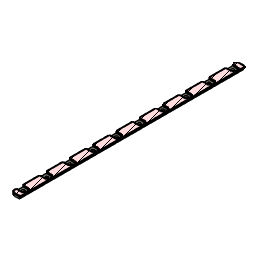
voron_v0_new_nut_holder (Autodesk Fusion 360 design; units mm, degrees)
Autodesk Fusion 360 part; units mm, degrees
sketch "Sketch1" plane through (0, 0, 0) normal (0, 0, 1) x (1, 0, 0)
  circle A0 centre (0, 0) radius 1.25
  line L0 (2.45, 0) -> (1.225, 2.1218)
  line L1 (1.225, 2.1218) -> (-1.225, 2.1218)
  line L2 (-1.225, 2.1218) -> (-2.45, 0) construction
  line L3 (-2.45, 0) -> (-1.225, -2.1218) construction
  line L4 (-1.225, -2.1218) -> (1.225, -2.1218)
  line L5 (1.225, -2.1218) -> (2.45, 0)
  line L6 (2.75, 223.4444) -> (2.75, -43.6896) construction
  line L7 (-2.75, 222.414) -> (-2.75, -48.8416) construction
  line L8 (-4.3569, -5.0218) -> (6.2765, -5.0218) construction
  line L9 (-4.4785, 139.9782) -> (4.5564, 139.9782) construction
  line L10 (-1.225, 2.1218) -> (-4.4593, 2.1218)
  line L11 (-1.225, -2.1218) -> (-4.4422, -2.1218)
  line L12 (-2.75, 139.9782) -> (2.75, 139.9782)
  line L13 (2.75, 139.9782) -> (2.75, -5.0218)
  line L14 (2.75, -5.0218) -> (-2.75, -5.0218)
  line L15 (-2.75, -5.0218) -> (-2.75, 139.9782)
  line L16 (-1.225, 17.1218) -> (-4.4593, 17.1218)
  line L17 (1.225, 17.1218) -> (-1.225, 17.1218)
  line L18 (2.45, 15) -> (1.225, 17.1218)
  line L19 (1.225, 12.8782) -> (2.45, 15)
  line L20 (-1.225, 12.8782) -> (1.225, 12.8782)
  line L21 (-1.225, 12.8782) -> (-4.4422, 12.8782)
  circle A1 centre (0, 15) radius 1.25
  line L22 (-1.225, 17.1218) -> (-2.45, 15) construction
  line L23 (-2.45, 15) -> (-1.225, 12.8782) construction
  line L24 (-1.225, 32.1218) -> (-4.4593, 32.1218)
  line L25 (1.225, 32.1218) -> (-1.225, 32.1218)
  line L26 (2.45, 30) -> (1.225, 32.1218)
  line L27 (1.225, 27.8782) -> (2.45, 30)
  line L28 (-1.225, 27.8782) -> (1.225, 27.8782)
  line L29 (-1.225, 27.8782) -> (-4.4422, 27.8782)
  circle A2 centre (0, 30) radius 1.25
  line L30 (-1.225, 32.1218) -> (-2.45, 30) construction
  line L31 (-2.45, 30) -> (-1.225, 27.8782) construction
  line L32 (-1.225, 47.1218) -> (-4.4593, 47.1218)
  line L33 (1.225, 47.1218) -> (-1.225, 47.1218)
  line L34 (2.45, 45) -> (1.225, 47.1218)
  line L35 (1.225, 42.8782) -> (2.45, 45)
  line L36 (-1.225, 42.8782) -> (1.225, 42.8782)
  line L37 (-1.225, 42.8782) -> (-4.4422, 42.8782)
  circle A3 centre (0, 45) radius 1.25
  line L38 (-1.225, 47.1218) -> (-2.45, 45) construction
  line L39 (-2.45, 45) -> (-1.225, 42.8782) construction
  line L40 (-1.225, 62.1218) -> (-4.4593, 62.1218)
  line L41 (1.225, 62.1218) -> (-1.225, 62.1218)
  line L42 (2.45, 60) -> (1.225, 62.1218)
  line L43 (1.225, 57.8782) -> (2.45, 60)
  line L44 (-1.225, 57.8782) -> (1.225, 57.8782)
  line L45 (-1.225, 57.8782) -> (-4.4422, 57.8782)
  circle A4 centre (0, 60) radius 1.25
  line L46 (-1.225, 62.1218) -> (-2.45, 60) construction
  line L47 (-2.45, 60) -> (-1.225, 57.8782) construction
  line L48 (-1.225, 77.1218) -> (-4.4593, 77.1218)
  line L49 (1.225, 77.1218) -> (-1.225, 77.1218)
  line L50 (2.45, 75) -> (1.225, 77.1218)
  line L51 (1.225, 72.8782) -> (2.45, 75)
  line L52 (-1.225, 72.8782) -> (1.225, 72.8782)
  line L53 (-1.225, 72.8782) -> (-4.4422, 72.8782)
  circle A5 centre (0, 75) radius 1.25
  line L54 (-1.225, 77.1218) -> (-2.45, 75) construction
  line L55 (-2.45, 75) -> (-1.225, 72.8782) construction
  line L56 (-1.225, 92.1218) -> (-4.4593, 92.1218)
  line L57 (1.225, 92.1218) -> (-1.225, 92.1218)
  line L58 (2.45, 90) -> (1.225, 92.1218)
  line L59 (1.225, 87.8782) -> (2.45, 90)
  line L60 (-1.225, 87.8782) -> (1.225, 87.8782)
  line L61 (-1.225, 87.8782) -> (-4.4422, 87.8782)
  circle A6 centre (0, 90) radius 1.25
  line L62 (-1.225, 92.1218) -> (-2.45, 90) construction
  line L63 (-2.45, 90) -> (-1.225, 87.8782) construction
  line L64 (-1.225, 107.1218) -> (-4.4593, 107.1218)
  line L65 (1.225, 107.1218) -> (-1.225, 107.1218)
  line L66 (2.45, 105) -> (1.225, 107.1218)
  line L67 (1.225, 102.8782) -> (2.45, 105)
  line L68 (-1.225, 102.8782) -> (1.225, 102.8782)
  line L69 (-1.225, 102.8782) -> (-4.4422, 102.8782)
  circle A7 centre (0, 105) radius 1.25
  line L70 (-1.225, 107.1218) -> (-2.45, 105) construction
  line L71 (-2.45, 105) -> (-1.225, 102.8782) construction
  line L72 (-1.225, 122.1218) -> (-4.4593, 122.1218)
  line L73 (1.225, 122.1218) -> (-1.225, 122.1218)
  line L74 (2.45, 120) -> (1.225, 122.1218)
  line L75 (1.225, 117.8782) -> (2.45, 120)
  line L76 (-1.225, 117.8782) -> (1.225, 117.8782)
  line L77 (-1.225, 117.8782) -> (-4.4422, 117.8782)
  circle A8 centre (0, 120) radius 1.25
  line L78 (-1.225, 122.1218) -> (-2.45, 120) construction
  line L79 (-2.45, 120) -> (-1.225, 117.8782) construction
  line L80 (-1.225, 137.1218) -> (-4.4593, 137.1218)
  line L81 (1.225, 137.1218) -> (-1.225, 137.1218)
  line L82 (2.45, 135) -> (1.225, 137.1218)
  line L83 (1.225, 132.8782) -> (2.45, 135)
  line L84 (-1.225, 132.8782) -> (1.225, 132.8782)
  line L85 (-1.225, 132.8782) -> (-4.4422, 132.8782)
  circle A9 centre (0, 135) radius 1.25
  line L86 (-1.225, 137.1218) -> (-2.45, 135) construction
  line L87 (-2.45, 135) -> (-1.225, 132.8782) construction
  dimension "d1" = 2.5
  dimension "d2" = 2.45
  dimension "d3" = 2.75
  dimension "d4" = 2.75
  dimension "d5" = 2.9
  dimension "d6" = 145
  dimension "d9" = 0
  dimension "d10" = 15
  dimension "d28" = 4.2435
  constraint coincident A0.centre origin
  constraint vertical L6
  constraint vertical L7
  constraint horizontal L8
  constraint horizontal L9
  constraint parallel L1 L10
  constraint perpendicular L7 L11
  constraint horizontal L12
  constraint vertical L13
  constraint horizontal L14
  constraint vertical L15
  constraint coincident L6 L13.end
  constraint coincident L8 L13.end
  constraint coincident L9 L12.start
  constraint coincident L7 L12.start
  measures "d1" diameter of A0
  measures "d2" distance of L0.start A0.centre
  measures "d3" distance of A0.centre L6
  measures "d4" distance of A0.centre L7
  measures "d5" distance of L4 L8
  measures "d6" distance of L8 L9
  measures "d28" distance of L10 L11
extrude "Extrude1" add sketch "Sketch1" along normal blind 0.8
extrude "Extrude2" add sketch "Sketch1" along normal blind 1.7 from surface at 0.8 contours L0 L1 L4 L5 L10 L11 L12 L13 L14 L15 L16 L17 L18 L19 L20 L21 L24 L25 L26 L27 L28 L29 L32 L33 L34 L35 L36 L37 L40 L41 L42 L43 L44 L45 L48 L49 L50 L51 L52 L53 L56 L57 L58 L59 L60 L61 L64 L65 L66 L67 L68 L69 L72 L73 L74 L75 L76 L77 L80 L81 L82 L83 L84 L85
sketch "Sketch3" plane through (0, -5.0218, 0) normal (0, -1, 0) x (1, 0, 0)
  line L0 (-2.75, 0) -> (2.75, 0)
  line L1 (2.75, 0) -> (2.75, 2.5)
  line L2 (2.75, 2.5) -> (-2.75, 2.5)
  line L3 (-2.75, 2.5) -> (-2.75, 0)
  line L4 (0, 2.5) -> (0, 4.2) construction
  line L5 (0, 4.2) -> (1.5, 4.2)
  line L6 (0, 4.2) -> (-1.5, 4.2)
  line L7 (-2.5489, 5.2) -> (3.0136, 5.2) construction
  line L8 (-2.75, 2.5) -> (-0.6708, 4.5792)
  line L9 (-2.75, 2.5) -> (0.1904, 2.5) construction
  line L10 (2.75, 2.5) -> (0.6708, 4.5792)
  dimension "d16" = 1.7
  dimension "d17" = 1.5
  dimension "d18" = 2.7
  dimension "d19" = 45
  constraint midpoint L2 L4.start
  constraint perpendicular L2 L4
  constraint perpendicular L4 L5
  constraint symmetric L5.start L4 L6.start
  constraint symmetric L4 L5.end L6.end
  constraint horizontal L7
  constraint horizontal L9
  constraint coincident L2.end L3.start
  constraint symmetric L4 L2.end L1.end
  constraint symmetric L4 L8.end L10.end
  measures "d16" distance of L4.start L4.end
  measures "d17" distance of L4.end L5.end
  measures "d18" distance of L2 L7
  measures "d19" angle of L8 L9
extrude "Extrude3" add sketch "Sketch3" against normal up to surface (145 mm away) contours L2 L5 L6 L8 L10
extrude "Extrude4" cut sketch "Sketch1" along normal blind 6.186 contours A0 | A1 | A2 | A3 | A4 | A5 | A6 | A7 | A8 | A9
chamfer "Chamfer1" distance 0.25 angle 45 4 edges at (2.75, 67.4782, 0) (2.75, 139.9782, 1.25) (2.75, -5.0218, 1.25) (2.75, 67.4782, 2.5)
fillet "Fillet1" radius 1.7 2 edges at (-2.75, 139.9782, 1.25) (-2.75, -5.0218, 1.25)
chamfer "Chamfer2" distance 0.4 angle 45 30 edges at (-2.75, 2.1218, 1.65) (-2.75, 0, 0.8) (-2.75, -2.1218, 1.65) (-2.75, 17.1218, 1.65) (-2.75, 15, 0.8) (-2.75, 12.8782, 1.65) (-2.75, 32.1218, 1.65) (-2.75, 30, 0.8) (-2.75, 27.8782, 1.65) (-2.75, 47.1218, 1.65) (-2.75, 45, 0.8) (-2.75, 42.8782, 1.65) (-2.75, 57.8782, 1.65) (-2.75, 60, 0.8) (-2.75, 62.1218, 1.65) (-2.75, 75, 0.8) (-2.75, 72.8782, 1.65) (-2.75, 77.1218, 1.65) (-2.75, 87.8782, 1.65) (-2.75, 90, 0.8) (-2.75, 92.1218, 1.65) (-2.75, 107.1218, 1.65) (-2.75, 105, 0.8) (-2.75, 102.8782, 1.65) (-2.75, 117.8782, 1.65) (-2.75, 120, 0.8) (-2.75, 122.1218, 1.65) (-2.75, 132.8782, 1.65) (-2.75, 135, 0.8) (-2.75, 137.1218, 1.65)
sketch "Sketch4" plane through (0, 0, 0) normal (0, 0, -1) x (1, 0, 0)
  circle A0 centre (0, -135) radius 1.25
  circle A1 centre (0, -120) radius 1.25
  circle A2 centre (0, -105) radius 1.25
  circle A3 centre (0, -90) radius 1.25
  circle A4 centre (0, -75) radius 1.25
  circle A5 centre (0, -60) radius 1.25
  circle A6 centre (0, -45) radius 1.25
  circle A7 centre (0, -30) radius 1.25
  circle A8 centre (0, -15) radius 1.25
  circle A9 centre (0, 0) radius 1.25
  arc A10 (-1.05, 5.0218) -> (-2.75, 3.3218) centre (-1.05, 3.3218) ccw
  line L0 (-2.75, 3.3218) -> (-2.75, -138.2782)
  arc A11 (-2.75, -138.2782) -> (-1.05, -139.9782) centre (-1.05, -138.2782) ccw
  line L1 (-1.05, -139.9782) -> (2.5, -139.9782)
  line L2 (2.5, -139.9782) -> (2.5, 5.0218)
  line L3 (2.5, 5.0218) -> (-1.05, 5.0218)
  circle A12 centre (0, 0) radius 0.9
  circle A13 centre (0, -15) radius 0.9
  circle A14 centre (0, -30) radius 0.9
  circle A15 centre (0, -45) radius 0.9
  circle A16 centre (0, -60) radius 0.9
  circle A17 centre (0, -75) radius 0.9
  circle A18 centre (0, -90) radius 0.9
  circle A19 centre (0, -105) radius 0.9
  circle A20 centre (0, -120) radius 0.9
  circle A21 centre (0, -135) radius 0.9
  dimension "d29" = 1.8
  dimension "d32" = 0
  dimension "d33" = -15
  constraint concentric A9 A12
  measures "d29" diameter of A12
extrude "Extrude5" add sketch "Sketch4" against normal up to surface (0.8 mm away) contours A0 | A1 | A2 | A3 | A4 | A5 | A6 | A7 | A8 | A9
equation "d2 = ( 4.9 / 2 ) * 1 mm"
equation "d3 = ( 5.5 / 2 ) * 1 mm"
equation "d4 = ( 5.5 / 2 ) * 1 mm"
